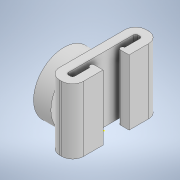
# Autodesk Inventor part: FS-01-SLBV2
Saved by Autodesk Inventor 2022.2 (Build 262287000, 287)
## iProperties
Created: 2021-12-12
Part Number: FS-01-SLBV2
Material: Generic
Document SubType Name: Modeling
Designer: Frank
Density: 1 g/cm^3
Appearance: Default
Author: Frank
Autodesk Inventor part; units mm, degrees
ref_plane "YZ Plane" through (0, 0, 0) normal (1, 0, 0) x (0, 1, 0)
ref_plane "XZ Plane" through (0, 0, 0) normal (0, 1, 0) x (-1, 0, 0)
ref_plane "XY Plane" through (0, 0, 0) normal (0, 0, 1) x (1, 0, 0)
sketch "Sketch1" plane through (0, 0, 0) normal (0, 1, 0) x (-1, 0, 0)
  line L0 (-0.25, 8) -> (0.25, 8)
  line L1 (0.75, 7.5) -> (0.75, -7.5)
  line L2 (0.25, -8) -> (-0.25, -8)
  line L3 (-0.75, -7.5) -> (-0.75, 7.5)
  line L4 (-0.75, 8) -> (0.75, -8) construction
  line L5 (0.75, 8) -> (-0.75, -8) construction
  arc A0 (0.25, -8) -> (0.75, -7.5) centre (0.25, -7.5) ccw
  arc A1 (-0.75, -7.5) -> (-0.25, -8) centre (-0.25, -7.5) ccw
  arc A2 (-0.25, 8) -> (-0.75, 7.5) centre (-0.25, 7.5) ccw
  arc A3 (0.75, 7.5) -> (0.25, 8) centre (0.25, 7.5) ccw
  line L6 (-0.25, -10) -> (0.25, -10)
  arc A4 (0.25, -10) -> (2.75, -7.5) centre (0.25, -7.5) ccw
  line L7 (2.75, -7.5) -> (2.75, 7.5)
  arc A5 (2.75, 7.5) -> (0.25, 10) centre (0.25, 7.5) ccw
  line L8 (0.25, 10) -> (-0.25, 10)
  arc A6 (-0.25, 10) -> (-2.75, 7.5) centre (-0.25, 7.5) ccw
  line L9 (-2.75, 7.5) -> (-2.75, -7.5)
  arc A7 (-2.75, -7.5) -> (-0.25, -10) centre (-0.25, -7.5) ccw
  line L10 (-0.75, 3) -> (-2.75, 3)
  line L11 (-0.75, -3) -> (-2.75, -3)
  line L12 (2.75, 0) -> (-2.75, 0) construction
  arc A8 (-0.75, -4) -> (-0.75, -3) centre (-0.75, -3.5) ccw
  arc A9 (-0.75, 3) -> (-0.75, 4) centre (-0.75, 3.5) ccw
  point P0 (0, 0)
  point P1 (0, 8)
  point P2 (-1.75, -3)
  dimension "d0" = 0.5
  dimension "d2" = 2
  dimension "d3" = 16
  dimension "d4" = 1.5
  dimension "d5" = 6
  dimension "d19" = 0.5
  constraints: 26 end point, 20 point on circle, 14 point on line, 10 centre point, 10 tangent, 6 midpoint, 5 parallel, 4 equal radius, 3 perpendicular, 1 horizontal, 8 other
  measures "d0" radius of A0
  measures "d2" distance between parallel lines of L2 L6
  measures "d3" distance from line of L2 point (0, 8)
  measures "d4" distance between parallel lines of L1 L3
  measures "d5" distance from line of point (-1.75, -3) L10
  measures "d19" radius of A8
extrude "Extrusion1" add sketch "Sketch1" along normal mid plane 15 contours A2 L3 L10 L9 A6 L8 A5 L7 A4 L6 A7 L11 A1 L2 A0 L1 A3 L0 | A9 L3 | A8 L3
sketch "Sketch2" plane through (0, 0, 0) normal (0, 0, 1) x (1, 0, 0)
  line L0 (-2.75, -2.5) -> (-9.25, -2.5)
  line L1 (-9.25, -2.5) -> (-9.25, -9.5)
  line L2 (-9.25, -9.5) -> (-5.25, -9.5)
  line L3 (-5.25, -9.5) -> (-5.25, -7.5)
  line L4 (-5.25, -7.5) -> (-2.75, -7.5)
  line L5 (-0.75, -7.5) -> (-2.75, -7.5) projected
  line L6 (-2.75, -7.5) -> (-2.75, 7.5) projected
  line L7 (-2.75, 7.5) -> (-0.75, 7.5) projected
  line L8 (-0.75, 7.5) -> (-0.75, -7.5) projected
  point P0 (0, 0)
  point P1 (-4, -7.5)
  point P2 (-5.25, -8.5)
  dimension "d8" = 14
  dimension "d9" = 10
  dimension "d10" = 2.5
  dimension "d11" = 6.5
  constraints: 10 end point, 3 perpendicular, 2 midpoint, 1 horizontal, 1 point on line, 1 vertical
  measures "d8" diameter of L2 L0
  measures "d9" diameter of point (-4, -7.5) L0
  measures "d10" distance from line of L6 point (-5.25, -8.5)
  measures "d11" distance from line of L0.start L1
revolve "Revolution1" add sketch "Sketch2" angle 360 about axis through (-2.75, -2.5, 0) along (-1, 0, 0) contours L6 L4 L3 L2 L1 L0
sketch "Sketch6" plane through (0, -7.5, 0) normal (0, -1, 0) x (1, 0, 0)
  point P0 (0, 0)
sketch "Sketch3" plane through (-9.25, -2.5, 0) normal (-1, 0, 0) x (0, 0, 1)
  circle A0 centre (0, 0) radius 7 projected
  line L0 (0, -5) -> (-7.5, -5) projected
  line L1 (7.5, -5) -> (0, -5) projected
  point P0 (0, 2.5)
  point P1 (4.899, -5)
  point P2 (-4.899, -5)
sketch "Sketch5" plane through (2.75, -7.5, 7.5) normal (1, 0, 0) x (0, 0, -1)
  circle A0 centre (7.5, 5) radius 5 projected
  point P0 (7.5, 7.5)
  point P1 (7.5, 0)
  constraints: 1 coincident, 1 vertical alignment
sketch "Sketch4" plane through (-9.25, -2.5, 0) normal (-1, 0, 0) x (0, 0, 1)
  point P0 (0, 2.5)
  point P1 (-0.0228, 0.0816)
body "Solid1"
